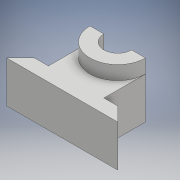
# Autodesk Inventor part: 01
Saved by Autodesk Inventor 2019 (Build 230136000, 136)
## iProperties
Created: 2020-09-23
Part Number: 01
Material: Generic
Document SubType Name: Modeling
Designer: USER
Density: 1 g/cm^3
Appearance: Default
Author: USER
Autodesk Inventor part; units mm, degrees
ref_plane "YZ Plane" through (0, 0, 0) normal (1, 0, 0) x (0, 1, 0)
ref_plane "XZ Plane" through (0, 0, 0) normal (0, 1, 0) x (-1, 0, 0)
ref_plane "XY Plane" through (0, 0, 0) normal (0, 0, 1) x (1, 0, 0)
sketch "草圖1" plane through (0, 0, 0) normal (0, 0, 1) x (1, 0, 0)
  line L0 (-20, 0) -> (20, 0)
  line L1 (20, 0) -> (20, -40)
  line L2 (20, -40) -> (-20, -40)
  line L3 (-20, -40) -> (-20, 0)
  line L4 (-20, -40) -> (-40, -40)
  line L5 (-40, -40) -> (-40, -30)
  line L6 (-40, -30) -> (-20, -30)
  line L7 (-20, -30) -> (-20, -40)
  line L8 (20, -40) -> (40, -40)
  line L9 (40, -40) -> (40, -30)
  line L10 (40, -30) -> (20, -30)
  line L11 (20, -30) -> (20, -40)
  point P0 (0, 0)
  point P1 (0, 0)
  dimension "d14" = 10
  dimension "d0" = 40
  dimension "d1" = 40
  dimension "d2" = 20
  dimension "d3" = 20
  dimension "d4" = 10
  constraints: 24 end point, 6 parallel, 3 horizontal, 3 perpendicular, 2 coincident, 1 horizontal alignment, 1 midpoint, 1 point on line
  measures "d0" distance of L1.end L2.end
  measures "d1" distance of L0.end L1.end
  measures "d2" distance of L2.end L4.end
  measures "d3" distance of L1.end L8.end
  measures "d4" distance of L4.end L5.end
extrude "擠出1" add sketch "草圖1" against normal blind 30
sketch "草圖2" plane through (0, 0, 0) normal (0, 0, 1) x (1, 0, 0)
  line L0 (20, 0) -> (-20, 0) projected
  arc A0 (-20, 0) -> (20, 0) centre (0, 0) ccw
  dimension "d8" = 20
  constraints: 2 point on circle, 1 centre point
  measures "d8" radius of A0
extrude "擠出2" add sketch "草圖2" along normal blind 10
sketch "草圖3" plane through (0, 0, 10) normal (0, 0, 1) x (1, 0, 0)
  circle A0 centre (0, 0) radius 10
  dimension "d11" = 20
  constraints: 1 centre point, 1 coincident
  measures "d11" diameter of A0
extrude "擠出3" cut sketch "草圖3" against normal through all
chamfer "倒角1" distance 10 angle 45 2 edges at (40, -30, -15) (-40, -30, -15)
equation "\"d14\" = 0.25 * d0"
equation "\"d1\" = d0"
equation "\"d2\" = 0.5 * d0"
equation "\"d3\" = 0.5 * d0"
equation "\"d4\" = 0.25 * d0"
equation "\"d5\" = 0.75 * d0"
equation "\"d8\" = 0.5 * d0"
equation "\"d9\" = 0.25 * d0"
equation "\"d11\" = 0.5 * d0"
